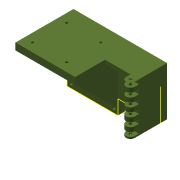
# Autodesk Inventor part: cellSTORM_cellphone_objectivelens_mount
Saved by Autodesk Inventor 2019 (Build 230136000, 136)
## iProperties
Created: 2019-10-29
Part Number: cellSTORM_cellphone_objectivelens_mount
Material: Generic
Document SubType Name: Modeling
Designer: diederichbenedict
Density: 1 g/cm^3
Appearance: Olive Green
Author: diederichbenedict
Autodesk Inventor part; units mm, degrees
ref_plane "YZ Plane" through (0, 0, 0) normal (1, 0, 0) x (0, 1, 0)
ref_plane "XZ Plane" through (0, 0, 0) normal (0, 1, 0) x (-1, 0, 0)
ref_plane "XY Plane" through (0, 0, 0) normal (0, 0, 1) x (1, 0, 0)
ref_plane "Work Plane1" through (0, 0, 0) normal (0, 0, 1) x (1, 0, 0)
sketch "Sketch1" plane through (0, 0, 0) normal (0, 0, 1) x (1, 0, 0)
  line L0 (28, 30) -> (30, 28) construction
  line L1 (28, 30) -> (-28, 30) construction
  line L2 (-30, 28) -> (-28, 30) construction
  line L3 (-30, 28) -> (-30, -28) construction
  line L4 (-28, -30) -> (-30, -28) construction
  line L5 (-28, -30) -> (28, -30) construction
  line L6 (30, -28) -> (28, -30) construction
  line L7 (30, -28) -> (30, 28) construction
  circle A0 centre (-17.5, -17.5) radius 1.95 projected
  circle A1 centre (17.5, 17.5) radius 1.95 projected
  circle A2 centre (17.5, -17.5) radius 1.95 projected
  circle A3 centre (-17.5, 17.5) radius 1.95 projected
  circle A4 centre (0, 0) radius 7.5 construction
  line L8 (-52.85, 44) -> (87.15, 44) construction
  line L9 (-30, -30) -> (30, -30)
  line L10 (30, -30) -> (30, 44)
  line L11 (30, 44) -> (-30, 44)
  line L12 (-30, 44) -> (-30, -30)
  line L13 (42.65, -13) -> (79.65, -13) construction
  line L14 (42.65, 36.7) -> (42.65, -13) construction
  line L15 (79.65, 36.7) -> (42.65, 36.7) construction
  line L16 (79.65, 36.7) -> (79.65, -13) construction
  line L17 (79.65, -13) -> (30, -13)
  line L18 (30, -13) -> (30, 23.9)
  line L19 (30, 23.9) -> (79.65, 23.9)
  line L20 (79.65, 23.9) -> (79.65, -13)
  line L21 (-15, -15) -> (15, -15)
  line L22 (15, -15) -> (15, 15)
  line L23 (15, 15) -> (-15, 15)
  line L24 (-15, 15) -> (-15, -15)
  line L25 (-15, -15) -> (15, 15) construction
  line L26 (15, -15) -> (-15, 15) construction
  circle A5 centre (48.55, -3.3) radius 4.5 projected
  circle A6 centre (61.15, 21.7) radius 4.5 projected
  circle A7 centre (73.75, -3.3) radius 4.5 projected
  line L27 (25, -25) -> (-25, -25) construction
  line L28 (-25, -25) -> (-25, 25) construction
  line L29 (-25, 25) -> (25, 25) construction
  line L30 (25, 25) -> (25, -25) construction
  line L31 (25, -25) -> (-25, 25) construction
  line L32 (-25, -25) -> (25, 25) construction
  circle A8 centre (-25, 25) radius 1.75
  circle A9 centre (25, 25) radius 1.75
  circle A10 centre (25, -25) radius 1.75
  circle A11 centre (-25, -25) radius 1.75
  point P0 (0, 0)
  dimension "d6" = 30
  dimension "d7" = 30
  dimension "d57" = 50
  dimension "d58" = 50
  dimension "d59" = 3.5
  dimension "d60" = 3.5
  dimension "d61" = 3.5
  dimension "d62" = 3.5
  constraints: 40 end point, 8 parallel, 4 centre point, 4 horizontal, 4 midpoint, 4 perpendicular, 3 coincident, 2 point on line
  measures "d6" distance of L23.end L22.end
  measures "d7" distance of L22.end L21.end
  measures "d57" distance of L28.end L29.end
  measures "d58" distance of L27.end L28.end
  measures "d59" diameter of A8
  measures "d60" diameter of A9
  measures "d61" diameter of A10
  measures "d62" diameter of A11
extrude "Extrusion1" add sketch "Sketch1" along normal blind 8 contours A0 | A1 | A2 | A3 | L12 L11 L10 L9 | L10 L19 A6 L20 L17 | L19 A6 | A5 | A7 picked at (60.9501, 21.68)
sketch "Sketch2" plane through (-30, 44, 0) normal (0, 1, 0) x (1, 0, 0)
  line L0 (60, 0) -> (60, -8) projected
  line L1 (0, 0) -> (0, -8) projected
  line L2 (60, -8) -> (0, -8) projected
  circle A0 centre (88.9869, -30.1976) radius 1.4 construction
  circle A1 centre (91.15, -56.0499) radius 15 construction
  line L3 (0, -8) -> (70, -8)
  line L4 (70, -8) -> (70, -68)
  line L5 (70, -68) -> (0, -68)
  line L6 (0, -68) -> (0, -8)
  point P0 (30, 0)
  dimension "d2" = 70
  dimension "d3" = 60
  constraints: 8 end point, 2 parallel, 1 horizontal, 1 perpendicular
  measures "d2" distance of L4.end L5.end
  measures "d3" distance of L3.end L4.end
extrude "Extrusion2" add sketch "Sketch2" against normal blind 8
sketch "Sketch3" plane through (0, 0, 8) normal (0, 0, 1) x (1, 0, 0)
  line L0 (30, 36) -> (-30, 36) projected
  line L1 (-30, 36) -> (-30, -30) projected
  line L2 (-30, -30) -> (30, -30) projected
  line L3 (30, -30) -> (30, -13) projected
  line L4 (30, -13) -> (79.65, -13) projected
  line L5 (79.65, -13) -> (79.65, 23.9) projected
  line L6 (79.65, 23.9) -> (30, 23.9) projected
  line L7 (30, 23.9) -> (30, 36) projected
  point P0 (0, 0)
sketch "Sketch4" plane through (-30, -30, 0) normal (-1, 0, 0) x (0, 0, 1)
  line L0 (0, 74) -> (0, 0) projected
  line L1 (0, 0) -> (8, 0) projected
  line L2 (8, 66) -> (8, 0) projected
  line L3 (68, 66) -> (8, 66) projected
  line L4 (68, 74) -> (68, 66) projected
  line L5 (0, 74) -> (68, 74) projected
  line L6 (68, 66) -> (8, 7.9065)
  line L7 (8, 53.9) -> (8, 66) projected
  line L8 (8, 7.9065) -> (8, 66)
  line L9 (8, 66) -> (68, 66) projected
  line L10 (8, 66) -> (68, 66)
  point P0 (0, 30)
  constraints: 6 end point, 1 perpendicular, 1 point on line, 1 vertical
extrude "Extrusion3" add sketch "Sketch4" against normal blind 4
pattern_linear "Rectangular Pattern1" count 2 spacing 56 along (1, 0, 0) of "Extrusion3"
sketch "Sketch7" plane through (30, 23.9, 0) normal (0, 1, 0) x (1, 0, 0)
  arc A0 (57.15, -64.5499) -> (60.65, -61.0499) centre (57.15, -61.0499) ccw projected
  line L0 (60.65, -2.1699) -> (60.65, -61.0499) projected
  arc A1 (60.65, -2.1699) -> (57.15, 1.3301) centre (57.15, -2.1699) ccw projected
  line L1 (-82.85, 1.3301) -> (57.15, 1.3301) projected
  arc A2 (-82.85, 1.3301) -> (-86.35, -2.1699) centre (-82.85, -2.1699) ccw projected
  line L2 (-86.35, -61.0499) -> (-86.35, -2.1699) projected
  arc A3 (-86.35, -61.0499) -> (-82.85, -64.5499) centre (-82.85, -61.0499) ccw projected
  line L3 (57.15, -64.5499) -> (-82.85, -64.5499) projected
  line L4 (49.65, 0) -> (49.65, -8) projected
  line L5 (49.65, -8) -> (39.65, -8)
  line L6 (39.65, -8) -> (39.65, -38)
  line L7 (39.65, -38) -> (49.65, -38) construction
  line L8 (49.65, -38) -> (49.65, -8)
  arc A4 (39.65, -38) -> (49.65, -38) centre (44.65, -38) ccw
  circle A5 centre (44.65, -38) radius 1.55
  point P0 (-30, 0)
  dimension "d25" = 10
  dimension "d26" = 30
  dimension "d27" = 3.1
  constraints: 8 end point, 2 centre point, 2 parallel, 2 point on circle, 2 tangent, 1 coincident, 1 horizontal, 1 perpendicular
  measures "d25" distance of L7.end L6.end
  measures "d26" distance of L6.end L5.end
  measures "d27" diameter of A5
extrude "Extrusion5" add sketch "Sketch7" along normal up to surface (57 mm away) from surface at -36.9 contours L8 A4 L6 L5
fillet "Fillet1" radius 10 1 edges at (69.65, 5.45, 8)
sketch "Sketch8" plane through (79.65, -13, 0) normal (1, 0, 0) x (0, 0, -1)
  line L0 (0, 0) -> (0, 36.9) projected
  line L1 (0, 36.9) -> (-8, 36.9) projected
  line L2 (-38, 0) -> (-38, 57) projected
  line L3 (0, 0) -> (-38, 0) projected
  line L4 (-38, 36.9) -> (-43, 36.9) projected
  line L5 (-43, 36.9) -> (-33, 36.9)
  line L6 (-33, 36.9) -> (-33, 31.9)
  line L7 (-33, 31.9) -> (-43, 31.9)
  line L8 (-43, 31.9) -> (-43, 36.9)
  line L9 (-8, 57) -> (-8, 36.9) projected
  line L10 (-8, 57) -> (-38, 57) projected
  point P0 (0, 13)
  dimension "d31" = 10
  dimension "d32" = 5
  constraints: 8 end point, 2 parallel, 1 horizontal, 1 perpendicular
  measures "d31" distance of L6.end L7.end
  measures "d32" distance of L5.end L6.end
extrude "Extrusion6" cut sketch "Sketch8" against normal up to surface (10 mm away) contours L7 L8 L4 L2 | L2 L5 L6 L7
pattern_linear "Rectangular Pattern2" count 6 spacing 10 along (0, -1, 0) count 3 spacing 10 along (0, 1, 0) of "Extrusion6"
sketch "Sketch9" plane through (0, 0, 0) normal (0, 0, -1) x (-1, 0, 0)
  line L0 (15, 15) -> (15, -15) projected
  line L1 (15, -15) -> (-15, -15) projected
  line L2 (-15, -15) -> (-15, 15) projected
  line L3 (-15, 15) -> (15, 15) projected
  line L4 (-79.65, -13) -> (-79.65, 23.9) projected
  line L5 (-30, -13) -> (-79.65, -13) projected
  line L6 (30, -30) -> (-30, -30) projected
  line L7 (30, 44) -> (30, -30) projected
  line L8 (-30, 44) -> (30, 44) projected
  line L9 (-79.65, 23.9) -> (-30, 23.9) projected
  circle A0 centre (-61.2, 5.45) radius 18.45 construction
  circle A1 centre (-61.2, 5.45) radius 6.3
  line L10 (-30, 23.9) -> (-30, 44) projected
  line L11 (-30, -30) -> (-30, -13) projected
  point P0 (0, 0)
  dimension "d38" = 12.6
  constraints: 3 tangent, 2 centre point, 1 coincident
  measures "d38" diameter of A1
extrude "Extrusion7" cut sketch "Sketch9" against normal blind 10 contours A1
sketch "Sketch10" plane through (0, 0, 8) normal (0, 0, 1) x (1, 0, 0)
  circle A0 centre (61.2, 5.45) radius 6.3 projected
  circle A1 centre (61.2, 5.45) radius 10.3
  point P0 (0, 0)
  dimension "d47" = 4
  constraints: 1 centre point
  measures "d47" radial gap between concentric circles of A0 A1
extrude "Extrusion8" add sketch "Sketch10" along normal blind 4
sketch "Sketch12" plane through (-30, 44, 0) normal (0, 1, 0) x (1, 0, 0)
  line L0 (60, 0) -> (0, 0) projected
  line L1 (0, 0) -> (0, -68) projected
  line L2 (70, -68) -> (0, -68) projected
  line L3 (70, -8) -> (70, -68) projected
  line L4 (60, -8) -> (70, -8) projected
  line L5 (60, 0) -> (60, -8) projected
  circle A0 centre (35, -33) radius 35
  line L6 (50, -58) -> (10, -58) construction
  line L7 (10, -58) -> (10, -18) construction
  line L8 (10, -18) -> (50, -18) construction
  line L9 (50, -18) -> (50, -58) construction
  line L10 (50, -58) -> (10, -18) construction
  line L11 (10, -58) -> (50, -18) construction
  point P0 (30, 0)
  point P1 (30, -38)
  dimension "d48" = 40
  dimension "d49" = 40
  constraints: 12 end point, 3 tangent, 2 midpoint, 2 parallel, 1 centre point, 1 horizontal, 1 perpendicular
  measures "d48" distance of L7.end L8.end
  measures "d49" distance of L6.end L7.end
hole "Hole2" at (-20, 44, 58) at (-20, 44, 18) at (20, 44, 58) at (20, 44, 18) direction (0, -1, 0) diameter 2.8 end through all
sketch "Sketch13" plane through (0, 0, 8) normal (0, 0, 1) x (1, 0, 0)
  arc A0 (-26, -26.4361) -> (-26, -23.5639) centre (-25, -25) ccw projected
  arc A1 (-26, 23.5639) -> (-26, 26.4361) centre (-25, 25) ccw projected
  arc A2 (26, 26.4361) -> (26, 23.5639) centre (25, 25) ccw projected
  arc A3 (26, -23.5639) -> (26, -26.4361) centre (25, -25) ccw projected
  point P0 (0, 0)
hole "Hole3" at (-25, -25, 8) at (-25, 25, 8) at (25, 25, 8) at (25, -25, 8) direction (0, 0, -1) diameter 3.9 depth 10 tip angle 118
sketch "Sketch14" plane through (0, 0, 8) normal (0, 0, 1) x (1, 0, 0)
  arc A0 (26, 26.6741) -> (26, 23.3259) centre (25, 25) ccw projected
  line L0 (26, 26.6741) -> (26, 36) projected
  line L1 (26, 36) -> (-26, 36) projected
  line L2 (-26, 36) -> (-26, 26.6741) projected
  arc A1 (-26, 23.3259) -> (-26, 26.6741) centre (-25, 25) ccw projected
  line L3 (-26, 23.3259) -> (-26, -22.0935) projected
  line L4 (-26, -22.0935) -> (-30, -22.0935) projected
  line L5 (-30, -22.0935) -> (-30, -30) projected
  line L6 (-30, -30) -> (30, -30) projected
  line L7 (30, -30) -> (30, -22.0935) projected
  line L8 (30, -22.0935) -> (26, -22.0935) projected
  line L9 (26, -22.0935) -> (26, 23.3259) projected
  circle A2 centre (-25, -25) radius 1.95 projected
  circle A3 centre (25, -25) radius 1.95 projected
  line L10 (-15, -15) -> (-15, 15) projected
  line L11 (-15, 15) -> (15, 15) projected
  line L12 (15, 15) -> (15, -15) projected
  line L13 (15, -15) -> (-15, -15) projected
  circle A4 centre (-25, 25) radius 4
  arc A5 (26, 26.6741) -> (26, 23.3259) centre (25, 25) ccw projected
  circle A6 centre (25, 25) radius 4
  point P0 (0, 0)
  dimension "d70" = 8
  dimension "d71" = 8
  constraints: 2 centre point, 2 coincident
  measures "d70" diameter of A4
  measures "d71" diameter of A6
extrude "Extrusion10" cut sketch "Sketch14" along normal blind 14 contours L0 A6 L9 A0 | A0 L9 A6 L0 | A4 L3 A1 L2 | L2 A1 L3 A4
sketch "Sketch15" plane through (30, 23.9, 0) normal (0, 1, 0) x (1, 0, 0)
  line L0 (49.65, 0) -> (49.65, -8) projected
  line L1 (49.65, 0) -> (0, 0) projected
  line L2 (0, -8) -> (0, 0) projected
  line L3 (29.65, -8) -> (0, -8) projected
  arc A0 (39.65, -18) -> (29.65, -8) centre (29.65, -18) ccw projected
  line L4 (39.65, -8) -> (39.65, -18) projected
  line L5 (49.65, -8) -> (39.65, -8) projected
  point P0 (-30, 0)
extrude "Extrusion11" add sketch "Sketch15" along normal up to surface (20.1 mm away)
sketch "Sketch16" plane through (-30, 44, 0) normal (0, 1, 0) x (1, 0, 0)
  line L0 (109.65, -33) -> (99.65, -33) projected
  line L1 (70, -8) -> (70, -68) projected
  line L2 (0, 0) -> (109.65, 0) projected
  line L3 (109.65, -33) -> (70, -33)
  line L4 (70, -33) -> (70, 0)
  line L5 (70, 0) -> (109.65, 0)
  line L6 (109.65, 0) -> (109.65, -33)
  point P0 (30, 0)
  constraints: 8 end point, 2 parallel, 1 horizontal, 1 perpendicular, 1 point on line
extrude "Extrusion12" add sketch "Sketch16" against normal blind 5
sketch "Sketch17" plane through (79.65, -13, 0) normal (1, 0, 0) x (0, 0, -1)
  line L0 (-33, 56.9) -> (-33, 51.9) projected
  line L1 (-33, 51.9) -> (-38, 51.9) projected
  line L2 (-38, 46.9) -> (-38, 51.9) projected
  line L3 (-38, 46.9) -> (-33, 46.9) projected
  line L4 (-33, 46.9) -> (-33, 41.9) projected
  line L5 (-33, 41.9) -> (-38, 41.9) projected
  line L6 (-38, 36.9) -> (-38, 41.9) projected
  line L7 (-38, 36.9) -> (-33, 36.9) projected
  line L8 (-33, 36.9) -> (-33, 31.9) projected
  line L9 (-33, 31.9) -> (-38, 31.9) projected
  line L10 (-38, 26.9) -> (-38, 31.9) projected
  line L11 (-38, 26.9) -> (-33, 26.9) projected
  line L12 (-33, 26.9) -> (-33, 21.9) projected
  line L13 (-33, 21.9) -> (-38, 21.9) projected
  line L14 (-38, 16.9) -> (-38, 21.9) projected
  line L15 (-38, 16.9) -> (-33, 16.9) projected
  line L16 (-33, 16.9) -> (-33, 11.9) projected
  line L17 (-33, 11.9) -> (-38, 11.9) projected
  line L18 (-38, 6.9) -> (-38, 11.9) projected
  line L19 (-38, 6.9) -> (-33, 6.9) projected
  line L20 (-33, 6.9) -> (-33, 1.9) projected
  line L21 (-33, 1.9) -> (-38, 1.9) projected
  line L22 (-38, 0) -> (-38, 1.9) projected
  line L23 (0, 0) -> (-38, 0) projected
  line L24 (0, 0) -> (0, 57) projected
  line L25 (0, 57) -> (-38, 57) projected
  line L26 (-38, 56.9) -> (-38, 57) projected
  line L27 (-38, 56.9) -> (-33, 56.9) projected
  line L28 (-33, 56.9) -> (-33, 51.9) projected
  line L29 (-33, 51.9) -> (-38, 51.9)
  line L30 (-38, 51.9) -> (-38, 57.6693)
  line L31 (-38, 57.6693) -> (-33, 57.6693)
  line L32 (-33, 57.6693) -> (-33, 51.9)
  line L33 (-32.2207, 6.9) -> (-43.7781, 6.9)
  line L34 (-43.7781, 6.9) -> (-43.7781, -2.7729)
  line L35 (-43.7781, -2.7729) -> (-32.2207, -2.7729)
  line L36 (-32.2207, -2.7729) -> (-32.2207, 6.9)
  line L37 (-33, 51.9) -> (-45.418, 51.9)
  line L38 (-45.418, 51.9) -> (-45.418, 59.4654)
  line L39 (-45.418, 59.4654) -> (-33, 59.4654)
  line L40 (-33, 59.4654) -> (-33, 51.9)
  point P0 (0, 13)
  constraints: 24 end point, 6 parallel, 3 horizontal, 3 perpendicular
extrude "Extrusion13" cut sketch "Sketch17" against normal up to surface (10 mm away) contours L0 L1 L30 L27 | L27 L26 L25 L32 | L30 L37 L38 L39 L40 L31 L26 | L25 L30 L31 L32 | L36 L35 L34 L33 L19 L20 L21 L22 L23 | L23 L22 L21 L20 L33 L36
body "Solid1"
